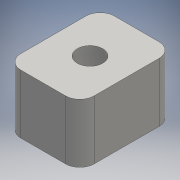
# Autodesk Inventor part: платик под двигатель
Saved by Autodesk Inventor 2016 (Build 200138000, 138)
## iProperties
Created: 2021-05-08
Part Number: платик под двигатель
Material: Типовые
Document SubType Name: Modeling
Designer: Лол
Density: 1 g/cm^3
Appearance: По умолчанию
Author: Лол
Autodesk Inventor part; units mm, degrees
ref_plane "YZ Plane" through (0, 0, 0) normal (1, 0, 0) x (0, 1, 0)
ref_plane "XZ Plane" through (0, 0, 0) normal (0, 1, 0) x (-1, 0, 0)
ref_plane "XY Plane" through (0, 0, 0) normal (0, 0, 1) x (1, 0, 0)
sketch "Эскиз1" plane through (0, 0, 0) normal (0, 0, 1) x (1, 0, 0)
  line L0 (18, -23) -> (-18, -23)
  line L1 (-18, -23) -> (-18, 23)
  line L2 (-18, 23) -> (18, 23)
  line L3 (18, 23) -> (18, -23)
  line L4 (18, -23) -> (-18, 23) construction
  line L5 (-18, -23) -> (18, 23) construction
  circle A0 centre (0, 0) radius 6.25
  dimension "d0" = 46
  dimension "d1" = 12.5
  dimension "d11" = 36
  constraints: 12 end point, 2 midpoint, 2 parallel, 1 centre point, 1 coincident, 1 horizontal, 1 perpendicular
  measures "d0" distance of L2.end L0.start
  measures "d1" diameter of A0
  measures "d11" distance between parallel lines of L1 L3
extrude "Выдавливание1" add sketch "Эскиз1" along normal blind 29
fillet "Сопряжение1" radius 7 4 edges at (-18, -23, 14.5) (-18, 23, 14.5) (18, 23, 14.5) (18, -23, 14.5)
sketch "Эскиз2" plane through (0, 0, 0) normal (0, 0, -1) x (-1, 0, 0)
  line L0 (-11, -23) -> (11, -23) projected
  line L1 (11, 23) -> (-11, 23) projected
  line L2 (-18, 16) -> (-18, -16) projected
  arc A0 (-18, -16) -> (-11, -23) centre (-11, -16) ccw projected
  arc A1 (11, -23) -> (18, -16) centre (11, -16) ccw projected
  arc A2 (18, 16) -> (11, 23) centre (11, 16) ccw projected
  arc A3 (-11, 23) -> (-18, 16) centre (-11, 16) ccw projected
  line L3 (18, -16) -> (18, 16) projected
  line L4 (-13, 18) -> (13, 18)
  line L5 (13, 18) -> (13, -18)
  line L6 (13, -18) -> (-13, -18)
  line L7 (-13, -18) -> (-13, 18)
  line L8 (-13, 18) -> (13, -18) construction
  line L9 (13, 18) -> (-13, -18) construction
  point P0 (0, 0)
  dimension "d12" = 5
  dimension "d13" = 5
  constraints: 12 end point, 2 midpoint, 2 parallel, 1 horizontal, 1 perpendicular
  measures "d12" distance between parallel lines of L0 L6
  measures "d13" distance between parallel lines of L3 L5
extrude "Выдавливание2" cut sketch "Эскиз2" against normal blind 5 contours L4 L5 L6 L7
fillet "Сопряжение3" radius 2 4 edges at (13, -18, 2.5) (-13, -18, 2.5) (-13, 18, 2.5) (13, 18, 2.5)
